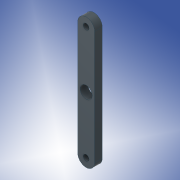
# Autodesk Inventor part: BearingCarrier
Saved by Autodesk Inventor 2017 SP1 (Build 210196100, 196)
## iProperties
Created: 2017-07-05
Part Number: BearingCarrier
Material: ABS Plastic
Document SubType Name: Modeling
Designer: zallen
Density: 1.06 g/cm^3
Appearance: CR Dark Blue
Author: zallen
Autodesk Inventor part; units mm, degrees
ref_plane "YZ Plane" through (0, 0, 0) normal (1, 0, 0) x (0, 1, 0)
ref_plane "XZ Plane" through (0, 0, 0) normal (0, 1, 0) x (-1, 0, 0)
ref_plane "XY Plane" through (0, 0, 0) normal (0, 0, 1) x (1, 0, 0)
sketch "Sketch1" plane through (0, 0, 0) normal (0, 0, 1) x (1, 0, 0)
  circle A0 centre (0, 0) radius 5.5 construction
  circle A1 centre (0, 74) radius 5.5 construction
  circle A2 centre (0, 74) radius 1.9
  circle A3 centre (0, 0) radius 1.9
  circle A4 centre (0, 37) radius 3.95
  line L0 (0, 74) -> (0, 0) construction
  line L1 (5.5, 74) -> (5.5, 0)
  line L2 (-5.5, 0) -> (-5.5, 74)
  arc A5 (5.5, 74) -> (-5.5, 74) centre (0, 74) ccw
  arc A6 (-5.5, 0) -> (5.5, 0) centre (0, 0) ccw
  dimension "d0" = 11
  dimension "d1" = 11
  dimension "d2" = 74
  dimension "d3" = 3.8
  dimension "d4" = 3.8
  dimension "d5" = 7.9
  constraints: 8 point on circle, 7 centre point, 6 end point, 6 tangent, 4 coincident, 2 vertical, 1 midpoint, 1 vertical alignment
  measures "d0" diameter of A0
  measures "d1" diameter of A1
  measures "d2" distance of point (0, 0) A1.centre
  measures "d3" diameter of A2
  measures "d4" diameter of A3
  measures "d5" diameter of A4
extrude "Extrusion1" add sketch "Sketch1" along normal blind 5
equation "\"d0\" = d1"
equation "\"d4\" = d3"
body "Solid1"
